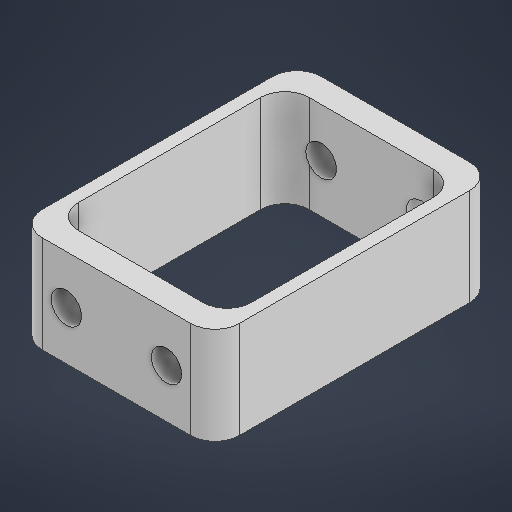
# Autodesk Inventor part: soporte inyector medio
Saved by Autodesk Inventor 2026.1 (Build 301233020, 233B)
## iProperties
Created: 2025-12-21
Part Number: soporte inyector medio
Material: Genérico
Document SubType Name: Modeling
Designer: patri
Density: 1 g/cm^3
Appearance: Valor por defecto
Author: patri
Autodesk Inventor part; units mm, degrees
ref_plane "YZ Plane" through (0, 0, 0) normal (1, 0, 0) x (0, 1, 0)
ref_plane "XZ Plane" through (0, 0, 0) normal (0, 1, 0) x (-1, 0, 0)
ref_plane "XY Plane" through (0, 0, 0) normal (0, 0, 1) x (1, 0, 0)
sketch "Boceto1" plane through (0, 0, 0) normal (0, 0, 1) x (1, 0, 0)
  line L0 (0, 0) -> (16.25, 0)
  line L1 (16.25, 0) -> (16.25, 8)
  line L2 (16.25, 8) -> (0, 8)
  line L3 (0, 8) -> (0, 0)
  line L4 (1, 8) -> (1, 0)
  line L5 (15.25, 8) -> (15.25, 0)
  circle A0 centre (4, 4) radius 1.25
  circle A1 centre (12.25, 4) radius 1.25
  point P0 (15.25, 4)
  point P1 (16.25, 4)
  point P2 (1, 4)
  point P3 (0, 4)
  dimension "d0" = 16.25
  dimension "d1" = 8
  dimension "d2" = 1
  dimension "d3" = 1
  dimension "d4" = 2.5
  dimension "d5" = 2.5
  dimension "d6" = 4
  dimension "d7" = 4
  dimension "d8" = 3
  dimension "d9" = 3
  constraints: 12 end point, 4 midpoint, 4 point on line, 3 perpendicular, 2 centre point, 2 parallel, 1 horizontal
  measures "d0" distance of L2.end L1.end
  measures "d1" distance of L1.end L0.end
  measures "d2" distance of point (15.25, 4) point (16.25, 4)
  measures "d3" distance of point (1, 4) point (0, 4)
  measures "d4" diameter of A0
  measures "d5" diameter of A1
  measures "d6" distance from line of L2 A1.centre
  measures "d7" distance from line of L2 A0.centre
  measures "d8" distance of point (15.25, 4) A1.centre
  measures "d9" distance from line of L4 A0.centre
extrude "Extrusión1" add sketch "Boceto1" along normal blind 23 contours L3 L2 L4 L0 | L5 L2 L1 L0
extrude "Extrusión2" add sketch "Boceto1" along normal blind 2 contours L4 L2 L5 L0
extrude "Extrusión3" add sketch "Boceto1" against normal blind 2 from surface at 23 contours L4 L2 L5 L0
fillet "Empalme1" radius 2 8 edges at (1, 4, 2) (15.25, 4, 2) (15.25, 4, 21) (16.25, 4, 23) (0, 4, 23) (1, 4, 21) (0, 4, 0) (16.25, 4, 0)
equation "\"d5\" = d4"
equation "\"d6\" = 0.5 * d1"
equation "\"d7\" = d6"
